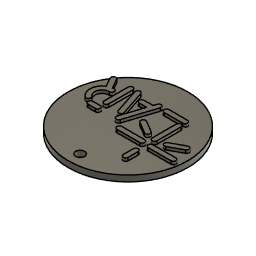
circle (Autodesk Fusion 360 design; units mm, degrees)
Autodesk Fusion 360 part; units mm, degrees
sketch "Esboço1" plane through (0, 0, 0) normal (0, 1, 0) x (1, 0, 0)
  circle A0 centre (0, 0) radius 20
  dimension "d1" = 40
  constraint coincident A0.centre origin
  measures "d1" diameter of A0
extrude "Extrusão1" add sketch "Esboço1" along normal blind 2
sketch "Esboço2" plane through (0, 2, 0) normal (0, 1, 0) x (-1, 0, 0)
  circle A0 centre (0, 0) radius 20
  arc A1 (-7.6957, 3.7284) -> (-7.6957, 2.0924) centre (-7.6957, 2.9104) ccw
  arc A2 (9.6001, 1.2824) -> (9.6001, -0.3536) centre (9.6001, 0.4644) ccw
  arc A3 (-8.3998, 9.9964) -> (-10.0358, 9.9964) centre (-9.2178, 9.9964) ccw
  arc A4 (12.1483, -0.3536) -> (12.1483, 1.2824) centre (12.1483, 0.4644) ccw
  arc A5 (-10.5289, 2.1733) -> (-10.5289, 3.8093) centre (-10.5289, 2.9913) ccw
  line L0 (4.3783, -2.0864) -> (7.1036, -10.37) construction
  line L1 (-10.0682, 0.3364) -> (-10.0682, -7.7023)
  line L2 (0.2484, -8.4101) -> (3.8683, -8.4101) construction
  line L3 (-7.6957, 2.9104) -> (-0.0057, 2.9104) construction
  line L4 (-10.0358, 9.9964) -> (-10.0358, 6.5964)
  line L5 (12.4242, -6.9719) -> (14.5369, -10.7718)
  line L6 (9.6001, -0.3536) -> (12.1483, -0.3536)
  line L7 (-8.3998, 6.5964) -> (-8.3998, 9.9964)
  line L8 (-9.2178, 9.9964) -> (-9.2178, 6.5964) construction
  line L9 (-13.1677, 0.533) -> (-17.5076, -1.7969)
  arc A6 (-9.2417, -9.0641) -> (-9.2417, -10.7001) centre (-9.2417, -9.8821) ccw
  line L10 (9.5376, -2.2788) -> (9.5376, -10.3735) construction
  line L11 (-10.5289, 3.8093) -> (-18.2117, 3.8093)
  line L12 (-9.2417, -10.7001) -> (-3.0317, -10.7001)
  arc A7 (-10.0358, 6.5964) -> (-8.3998, 6.5964) centre (-9.2178, 6.5964) ccw
  arc A8 (-12.3938, -0.9084) -> (-13.1677, 0.533) centre (-12.7808, -0.1877) ccw
  line L13 (0.5064, -10.266) -> (3.7944, -0.1298)
  line L14 (-7.6957, 2.0924) -> (-0.0057, 2.0924)
  line L15 (-0.0057, 3.7284) -> (-7.6957, 3.7284)
  arc A9 (-8.4322, 0.3364) -> (-10.0682, 0.3364) centre (-9.2502, 0.3364) ccw
  arc A10 (-0.0057, 2.0924) -> (-0.0057, 3.7284) centre (-0.0057, 2.9104) ccw
  arc A11 (3.7944, -0.1298) -> (2.2383, 0.375) centre (3.0163, 0.1226) ccw
  line L16 (12.1483, 1.2824) -> (9.6001, 1.2824)
  line L17 (0.2484, -9.2281) -> (3.8683, -9.2281)
  line L18 (-16.7338, -3.2383) -> (-12.3938, -0.9084)
  arc A12 (12.141, -6.7193) -> (14.2741, -1.032) centre (12.1819, -3.4909) ccw construction
  arc A13 (13.854, -6.1769) -> (12.4242, -6.9719) centre (13.1391, -6.5744) ccw
  arc A14 (14.5369, -10.7718) -> (15.9667, -9.9767) centre (15.2518, -10.3742) ccw
  line L19 (2.2383, 0.375) -> (-1.0498, -9.7612)
  arc A15 (5.1554, -1.8307) -> (3.6013, -2.342) centre (4.3783, -2.0864) ccw
  line L20 (9.6001, 0.4644) -> (12.1483, 0.4644) construction
  arc A16 (-17.5076, -1.7969) -> (-16.7338, -3.2383) centre (-17.1207, -2.5176) ccw
  line L21 (8.7196, -2.2788) -> (8.7196, -10.3735)
  line L22 (3.6013, -2.342) -> (6.3265, -10.6256)
  arc A17 (12.1514, -5.9012) -> (12.1306, -7.5373) centre (12.141, -6.7193) ccw
  arc A18 (12.1514, -5.9012) -> (13.7439, -1.6551) centre (12.1819, -3.4909) ccw
  arc A19 (-1.0498, -9.7612) -> (0.5064, -10.266) centre (-0.2717, -10.0136) ccw
  arc A20 (6.3265, -10.6256) -> (7.8806, -10.1144) centre (7.1036, -10.37) ccw
  arc A21 (3.8683, -9.2281) -> (3.8683, -7.5921) centre (3.8683, -8.4101) ccw
  line L23 (13.1391, -6.5744) -> (15.2518, -10.3742) construction
  arc A22 (12.1306, -7.5373) -> (14.8043, -0.4089) centre (12.1819, -3.4909) ccw
  line L24 (-6.0435, -0.6001) -> (-2.2156, -2.8491) construction
  line L25 (-6.4578, -1.3054) -> (-2.63, -3.5544)
  arc A23 (-3.0317, -10.7001) -> (-3.0317, -9.0641) centre (-3.0317, -9.8821) ccw
  arc A24 (10.3556, -2.2788) -> (8.7196, -2.2788) centre (9.5376, -2.2788) ccw
  line L26 (10.3556, -10.3735) -> (10.3556, -2.2788)
  line L27 (7.8806, -10.1144) -> (5.1554, -1.8307)
  line L28 (-1.8012, -2.1438) -> (-5.6291, 0.1051)
  arc A25 (0.2484, -7.5921) -> (0.2484, -9.2281) centre (0.2484, -8.4101) ccw
  line L29 (3.8683, -7.5921) -> (0.2484, -7.5921)
  arc A26 (-5.6291, 0.1051) -> (-6.4578, -1.3054) centre (-6.0435, -0.6001) ccw
  arc A27 (-2.63, -3.5544) -> (-1.8012, -2.1438) centre (-2.2156, -2.8491) ccw
  arc A28 (8.7196, -10.3735) -> (10.3556, -10.3735) centre (9.5376, -10.3735) ccw
  line L30 (-3.0317, -9.0641) -> (-9.2417, -9.0641)
  line L31 (-10.5289, 2.9913) -> (-18.2117, 2.9913) construction
  line L32 (-8.4322, -7.7023) -> (-8.4322, 0.3364)
  line L33 (-9.2417, -9.8821) -> (-3.0317, -9.8821) construction
  line L34 (-18.2117, 2.1733) -> (-10.5289, 2.1733)
  line L35 (15.9667, -9.9767) -> (13.854, -6.1769)
  line L36 (-17.1207, -2.5176) -> (-12.7808, -0.1877) construction
  arc A29 (-18.2117, 3.8093) -> (-18.2117, 2.1733) centre (-18.2117, 2.9913) ccw
  arc A30 (14.8043, -0.4089) -> (13.7439, -1.6551) centre (14.2741, -1.032) ccw
  line L37 (-0.2717, -10.0136) -> (3.0163, 0.1226) construction
  line L38 (-9.2502, 0.3364) -> (-9.2502, -7.7023) construction
  arc A31 (-10.0682, -7.7023) -> (-8.4322, -7.7023) centre (-9.2502, -7.7023) ccw
  point P0 (-1.3, 0)
  point P1 (-1.3, 0)
  point P2 (2.75, -13.35)
  point P3 (2.75, -13.35)
  point P4 (3.3879, -13.4686)
  point P5 (2.75, -13.35)
  point P6 (2.75, -13.35)
  point P7 (2.75, -13.35)
  dimension "d4" = 1.6362
  dimension "d5" = 1.636
  dimension "d6" = 1.636
  dimension "d7" = 1.636
  dimension "d8" = 1.636
  dimension "d9" = 1.636
  dimension "d10" = 1.636
  dimension "d11" = 1.636
  dimension "d12" = 1.636
  dimension "d13" = 4.4396
  dimension "d14" = 1.636
  dimension "d15" = 1.636
  dimension "d16" = 1.636
  dimension "d17" = 1.636
  dimension "d18" = 1.636
  dimension "d19" = 3.4
  constraint coincident P1 P0
  constraint tangent L4 A7
  constraint tangent L7 A7
  constraint parallel L4 L7
  constraint tangent A3 L7
  constraint tangent A3 L4
  constraint tangent L14 A10
  constraint tangent L15 A10
  constraint parallel L14 L15
  constraint tangent A1 L15
  constraint tangent A1 L14
  constraint tangent L25 A27
  constraint tangent L28 A27
  constraint parallel L25 L28
  constraint tangent L28 A26
  constraint tangent L25 A26
  constraint tangent L1 A31
  constraint tangent L32 A31
  constraint parallel L1 L32
  constraint tangent A9 L32
  constraint tangent L1 A9
  constraint tangent A8 L18
  constraint tangent L9 A8
  constraint parallel L9 L18
  constraint tangent L9 A16
  constraint tangent L18 A16
  constraint tangent L11 A29
  constraint tangent L34 A29
  constraint parallel L11 L34
  constraint tangent A5 L34
  constraint tangent A5 L11
  constraint perpendicular L1 L31
  constraint tangent L12 A23
  constraint tangent A23 L30
  constraint parallel L12 L30
  constraint tangent A6 L30
  constraint tangent A6 L12
  constraint perpendicular L1 L33
  constraint tangent L13 A11
  constraint tangent A11 L19
  constraint parallel L13 L19
  constraint tangent L19 A19
  constraint tangent L13 A19
  constraint tangent L17 A21
  constraint tangent A21 L29
  constraint parallel L17 L29
  constraint tangent A25 L29
  constraint tangent L17 A25
  constraint coincident L2.start L37
  constraint tangent L22 A20
  constraint tangent A20 L27
  constraint parallel L22 L27
  constraint tangent A15 L27
  constraint tangent A15 L22
  constraint tangent L21 A28
  constraint tangent L26 A28
  constraint parallel L21 L26
  constraint tangent A24 L26
  constraint tangent L21 A24
  constraint tangent A4 L6
  constraint tangent A4 L16
  constraint parallel L6 L16
  constraint tangent A2 L16
  constraint tangent A2 L6
  constraint tangent A17 A22
  constraint tangent A17 A18
  constraint tangent A18 A30
  constraint tangent A22 A30
  constraint tangent L5 A14
  constraint tangent A14 L35
  constraint parallel L5 L35
  constraint tangent A13 L35
  constraint tangent L5 A13
  constraint coincident A13.centre A12
  measures "d4" distance of A18 A22
  measures "d5" distance of L6 L16
  measures "d6" distance of L5 L35
  measures "d7" distance of L21 L26
  measures "d8" distance of L22 L27
  measures "d9" distance of L17 L29
  measures "d10" distance of L13 L19
  measures "d11" distance of L12 L30
  measures "d12" distance of L1 L32
  measures "d13" distance of L24.end L24.start
  measures "d14" distance of L25 L28
  measures "d15" distance of L14 L15
  measures "d16" distance of L11 L34
  measures "d17" distance of L4 L7
  measures "d18" distance of L9 L18
  measures "d19" distance of A3.centre L8.end
extrude "Extrusão2" add sketch "Esboço2" along normal blind 1 contours A1 L14 L15 A10 | A2 A4 L6 L16 | A3 L4 L7 A7 | A5 L11 L34 A29 | L1 A9 L32 A31 | L5 A13 A22 L35 | L5 A13 A17 A18 A22 | L5 A14 A22 L35 | A13 A18 A22 L35 A30 | L9 A8 L18 A16 | A6 L12 A23 L30 | L13 L17 L19 A19 A25 | L13 L17 A25 L29 | L13 L17 A21 L29 | L13 A11 L19 A25 L29 | A15 L22 A20 L27 | L21 A24 L26 A28 | L25 L28 A26 A27
sketch "Esboço3" plane through (0, 2, 0) normal (0, 1, 0) x (-1, 0, 0)
  arc A0 (12.1483, -0.3536) -> (12.1483, 1.2824) centre (12.1483, 0.4644) ccw
  line L0 (12.1483, -0.3536) -> (9.6001, -0.3536)
  arc A1 (9.6001, 1.2824) -> (9.6001, -0.3536) centre (9.6001, 0.4644) ccw
  line L1 (9.6001, 1.2824) -> (12.1483, 1.2824)
  arc A2 (3.8683, -9.2281) -> (3.8683, -7.5921) centre (3.8683, -8.4101) ccw
  line L2 (3.8683, -9.2281) -> (0.843, -9.2281)
  line L3 (0.843, -9.2281) -> (0.5064, -10.266)
  arc A3 (-1.0498, -9.7612) -> (0.5064, -10.266) centre (-0.2717, -10.0136) ccw
  line L4 (-1.0498, -9.7612) -> (2.2383, 0.375)
  arc A4 (3.7944, -0.1298) -> (2.2383, 0.375) centre (3.0163, 0.1226) ccw
  line L5 (3.7944, -0.1298) -> (1.3737, -7.5921)
  line L6 (1.3737, -7.5921) -> (3.8683, -7.5921)
  line L7 (-10.0682, -7.7023) -> (-10.0682, 0.3364)
  arc A5 (-8.4322, 0.3364) -> (-10.0682, 0.3364) centre (-9.2502, 0.3364) ccw
  line L8 (-8.4322, 0.3364) -> (-8.4322, -7.7023)
  arc A6 (-10.0682, -7.7023) -> (-8.4322, -7.7023) centre (-9.2502, -7.7023) ccw
  line L9 (-10.0358, 6.5964) -> (-10.0358, 9.9964)
  arc A7 (-8.3998, 9.9964) -> (-10.0358, 9.9964) centre (-9.2178, 9.9964) ccw
  line L10 (-8.3998, 9.9964) -> (-8.3998, 6.5964)
  arc A8 (-10.0358, 6.5964) -> (-8.3998, 6.5964) centre (-9.2178, 6.5964) ccw
  line L11 (-2.63, -3.5544) -> (-6.4578, -1.3054)
  arc A9 (-5.6291, 0.1051) -> (-6.4578, -1.3054) centre (-6.0435, -0.6001) ccw
  line L12 (-5.6291, 0.1051) -> (-1.8012, -2.1438)
  arc A10 (-2.63, -3.5544) -> (-1.8012, -2.1438) centre (-2.2156, -2.8491) ccw
  arc A11 (6.3265, -10.6256) -> (7.8806, -10.1144) centre (7.1036, -10.37) ccw
  line L13 (6.3265, -10.6256) -> (3.6013, -2.342)
  arc A12 (5.1554, -1.8307) -> (3.6013, -2.342) centre (4.3783, -2.0864) ccw
  line L14 (5.1554, -1.8307) -> (7.8806, -10.1144)
  arc A13 (12.1514, -5.9012) -> (13.7439, -1.6551) centre (12.1819, -3.4909) ccw
  arc A14 (14.8043, -0.4089) -> (13.7439, -1.6551) centre (14.2741, -1.032) ccw
  arc A15 (14.2834, -6.9492) -> (14.8043, -0.4089) centre (12.1819, -3.4909) ccw
  line L15 (14.2834, -6.9492) -> (15.9667, -9.9767)
  arc A16 (14.5369, -10.7718) -> (15.9667, -9.9767) centre (15.2518, -10.3742) ccw
  line L16 (14.5369, -10.7718) -> (12.7188, -7.5019)
  arc A17 (12.1306, -7.5373) -> (12.7188, -7.5019) centre (12.1819, -3.4909) ccw
  arc A18 (12.1514, -5.9012) -> (12.1306, -7.5373) centre (12.141, -6.7193) ccw
  arc A19 (-3.0317, -10.7001) -> (-3.0317, -9.0641) centre (-3.0317, -9.8821) ccw
  line L17 (-3.0317, -10.7001) -> (-9.2417, -10.7001)
  arc A20 (-9.2417, -9.0641) -> (-9.2417, -10.7001) centre (-9.2417, -9.8821) ccw
  line L18 (-9.2417, -9.0641) -> (-3.0317, -9.0641)
  line L19 (-17.5076, -1.7969) -> (-13.1677, 0.533)
  arc A21 (-12.3938, -0.9084) -> (-13.1677, 0.533) centre (-12.7808, -0.1877) ccw
  line L20 (-12.3938, -0.9084) -> (-16.7338, -3.2383)
  arc A22 (-17.5076, -1.7969) -> (-16.7338, -3.2383) centre (-17.1207, -2.5176) ccw
  line L21 (-18.2117, 3.8093) -> (-10.5289, 3.8093)
  arc A23 (-10.5289, 2.1733) -> (-10.5289, 3.8093) centre (-10.5289, 2.9913) ccw
  line L22 (-10.5289, 2.1733) -> (-18.2117, 2.1733)
  arc A24 (-18.2117, 3.8093) -> (-18.2117, 2.1733) centre (-18.2117, 2.9913) ccw
  line L23 (-0.0057, 2.0924) -> (-7.6957, 2.0924)
  arc A25 (-7.6957, 3.7284) -> (-7.6957, 2.0924) centre (-7.6957, 2.9104) ccw
  line L24 (-7.6957, 3.7284) -> (-0.0057, 3.7284)
  arc A26 (-0.0057, 2.0924) -> (-0.0057, 3.7284) centre (-0.0057, 2.9104) ccw
  line L25 (8.7196, -10.3735) -> (8.7196, -2.2788)
  arc A27 (10.3556, -2.2788) -> (8.7196, -2.2788) centre (9.5376, -2.2788) ccw
  line L26 (10.3556, -2.2788) -> (10.3556, -10.3735)
  arc A28 (8.7196, -10.3735) -> (10.3556, -10.3735) centre (9.5376, -10.3735) ccw
  circle A29 centre (0, 0) radius 20
  circle A30 centre (0, 16) radius 1.5
  dimension "d22" = 3
  measures "d22" diameter of A30
extrude "Extrusão3" cut sketch "Esboço3" against normal blind 6 contours A30
